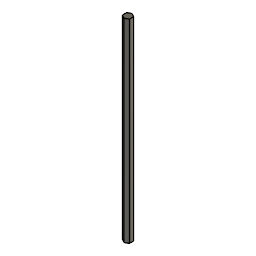
リアシャフト (Autodesk Fusion 360 design; units mm, degrees)
Autodesk Fusion 360 part; units mm, degrees
sketch "スケッチ1" plane through (0, 0, 0) normal (0, 0, 1) x (1, 0, 0)
  line L0 (1.299, -0.75) -> (1.299, 0.75)
  line L1 (1.299, 0.75) -> (0, 1.5)
  line L2 (0, 1.5) -> (-1.299, 0.75)
  line L3 (-1.299, 0.75) -> (-1.299, -0.75)
  line L4 (-1.299, -0.75) -> (0, -1.5)
  line L5 (0, -1.5) -> (1.299, -0.75)
  dimension "d1" = 1.5
  measures "d1" distance of L0.start origin
extrude "押し出し1" add sketch "スケッチ1" along normal blind 70
equation "d2 = 28 mm + ( 21 * 2 ) * 1 mm"
